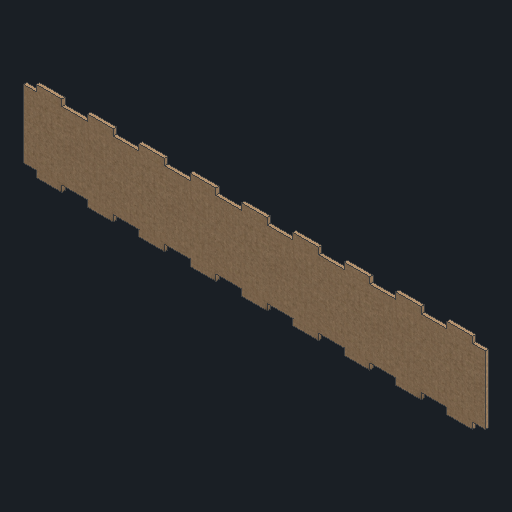
# Autodesk Inventor part: MainArmCenter
Saved by Autodesk Inventor 2024.1 (Build 281209000, 209)
## iProperties
Created: 2023-10-16
Part Number: MainArmCenter
Material: MDF Medium Density Fiberboard
Document SubType Name: Modeling
Designer: Brandon
Density: 0.8 g/cm^3
Appearance: Cardboard - Corrugated
Author: Brandon
Autodesk Inventor part; units mm, degrees
ref_plane "YZ Plane" through (0, 0, 0) normal (1, 0, 0) x (0, 1, 0)
ref_plane "XZ Plane" through (0, 0, 0) normal (0, 1, 0) x (-1, 0, 0)
ref_plane "XY Plane" through (0, 0, 0) normal (0, 0, 1) x (1, 0, 0)
sketch "Sketch1" plane through (0, 0, 0) normal (0, 0, 1) x (1, 0, 0)
  line L0 (-67.6755, -67.3) -> (481.6646, -67.3) projected
  line L1 (-67.6755, 0) -> (481.6646, 0) projected
  line L2 (0, 0) -> (25.4, 0)
  line L3 (25.4, 0) -> (25.4, 6.35)
  line L4 (25.4, 6.35) -> (0, 6.35)
  line L5 (0, 6.35) -> (0, 0)
  line L6 (0, -67.3) -> (25.4, -67.3)
  line L7 (25.4, -67.3) -> (25.4, -73.65)
  line L8 (25.4, -73.65) -> (0, -73.65)
  line L9 (0, -73.65) -> (0, -67.3)
  line L10 (50.8, -67.3) -> (76.2, -67.3)
  line L11 (76.2, -67.3) -> (76.2, -73.65)
  line L12 (76.2, -73.65) -> (50.8, -73.65)
  line L13 (50.8, -73.65) -> (50.8, -67.3)
  line L14 (50.8, 0) -> (76.2, 0)
  line L15 (76.2, 0) -> (76.2, 6.35)
  line L16 (76.2, 6.35) -> (50.8, 6.35)
  line L17 (50.8, 6.35) -> (50.8, 0)
  line L18 (101.6, -67.3) -> (127, -67.3)
  line L19 (127, -67.3) -> (127, -73.65)
  line L20 (127, -73.65) -> (101.6, -73.65)
  line L21 (101.6, -73.65) -> (101.6, -67.3)
  line L22 (101.6, 0) -> (127, 0)
  line L23 (127, 0) -> (127, 6.35)
  line L24 (127, 6.35) -> (101.6, 6.35)
  line L25 (101.6, 6.35) -> (101.6, 0)
  line L26 (152.4, -67.3) -> (177.8, -67.3)
  line L27 (177.8, -67.3) -> (177.8, -73.65)
  line L28 (177.8, -73.65) -> (152.4, -73.65)
  line L29 (152.4, -73.65) -> (152.4, -67.3)
  line L30 (152.4, 0) -> (177.8, 0)
  line L31 (177.8, 0) -> (177.8, 6.35)
  line L32 (177.8, 6.35) -> (152.4, 6.35)
  line L33 (152.4, 6.35) -> (152.4, 0)
  line L34 (203.2, -67.3) -> (228.6, -67.3)
  line L35 (228.6, -67.3) -> (228.6, -73.65)
  line L36 (228.6, -73.65) -> (203.2, -73.65)
  line L37 (203.2, -73.65) -> (203.2, -67.3)
  line L38 (203.2, 0) -> (228.6, 0)
  line L39 (228.6, 0) -> (228.6, 6.35)
  line L40 (228.6, 6.35) -> (203.2, 6.35)
  line L41 (203.2, 6.35) -> (203.2, 0)
  line L42 (254, -67.3) -> (279.4, -67.3)
  line L43 (279.4, -67.3) -> (279.4, -73.65)
  line L44 (279.4, -73.65) -> (254, -73.65)
  line L45 (254, -73.65) -> (254, -67.3)
  line L46 (254, 0) -> (279.4, 0)
  line L47 (279.4, 0) -> (279.4, 6.35)
  line L48 (279.4, 6.35) -> (254, 6.35)
  line L49 (254, 6.35) -> (254, 0)
  line L50 (304.8, -67.3) -> (330.2, -67.3)
  line L51 (330.2, -67.3) -> (330.2, -73.65)
  line L52 (330.2, -73.65) -> (304.8, -73.65)
  line L53 (304.8, -73.65) -> (304.8, -67.3)
  line L54 (304.8, 0) -> (330.2, 0)
  line L55 (330.2, 0) -> (330.2, 6.35)
  line L56 (330.2, 6.35) -> (304.8, 6.35)
  line L57 (304.8, 6.35) -> (304.8, 0)
  line L58 (355.6, -67.3) -> (381, -67.3)
  line L59 (381, -67.3) -> (381, -73.65)
  line L60 (381, -73.65) -> (355.6, -73.65)
  line L61 (355.6, -73.65) -> (355.6, -67.3)
  line L62 (355.6, 0) -> (381, 0)
  line L63 (381, 0) -> (381, 6.35)
  line L64 (381, 6.35) -> (355.6, 6.35)
  line L65 (355.6, 6.35) -> (355.6, 0)
  line L66 (406.4, -67.3) -> (431.8, -67.3)
  line L67 (431.8, -67.3) -> (431.8, -73.65)
  line L68 (431.8, -73.65) -> (406.4, -73.65)
  line L69 (406.4, -73.65) -> (406.4, -67.3)
  line L70 (406.4, 0) -> (431.8, 0)
  line L71 (431.8, 0) -> (431.8, 6.35)
  line L72 (431.8, 6.35) -> (406.4, 6.35)
  line L73 (406.4, 6.35) -> (406.4, 0)
  line L74 (444.5, -67.3) -> (444.5, 0)
  line L75 (-12.7, -67.3) -> (-12.7, 0)
  point P0 (25.4, -67.3)
  point P1 (50.8, -67.3)
  point P2 (76.2, -67.3)
  point P3 (101.6, -67.3)
  point P4 (127, -67.3)
  point P5 (152.4, -67.3)
  point P6 (177.8, -67.3)
  point P7 (203.2, -67.3)
  point P8 (228.6, -67.3)
  point P9 (254, -67.3)
  point P10 (279.4, -67.3)
  point P11 (304.8, -67.3)
  point P12 (330.2, -67.3)
  point P13 (355.6, -67.3)
  point P14 (381, -67.3)
  point P15 (406.4, -67.3)
  point P16 (431.8, -67.3)
  dimension "d0" = 25.4
  dimension "d1" = 6.35
  dimension "d2" = 25.4
  dimension "d3" = 6.35
  dimension "d6" = 50.8
  dimension "d11" = 12.7
  dimension "d12" = 12.7
  constraints: 148 end point, 64 horizontal alignment, 36 parallel, 32 collinear, 9 point on line, 2 horizontal, 2 perpendicular, 2 vertical, 7 other
  measures "d0" distance of L4.end L3.end
  measures "d1" distance of L3.end L2.end
  measures "d2" distance of L7.end L8.end
  measures "d3" distance of L6.end L7.end
  measures "d6" distance of L6.start L10.start
  measures "d11" distance between parallel lines of L75 L9
  measures "d12" distance between parallel lines of L67 L74
extrude "Extrusion1" add sketch "Sketch1" along normal blind 3.175
body "Solid1"
